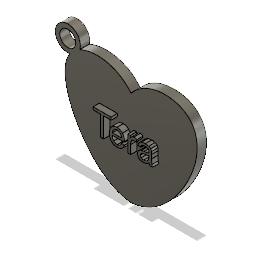
心挂件 (Autodesk Fusion 360 design; units mm, degrees)
Autodesk Fusion 360 part; units mm, degrees
sketch "草图15" plane through (0, 0, 0) normal (0, 0, 1) x (1, 0, 0)
  spline S0 degree 5 poles (0, 25) (-0.3399, 25.4215) (-1.0493, 26.2218) (-2.2021, 27.2937) (-3.9173, 28.4651) (-6.346, 29.4886) (-9.0135, 30.049) (-11.8244, 30.1104) (-14.6065, 29.6188) (-17.1328, 28.5147) (-19.1721, 26.7575) (-20.5275, 24.3447) (-21.0876, 21.3391) (-20.8505, 17.8796) (-19.8871, 14.1498) (-18.3175, 10.3575) (-16.2836, 6.7096) (-13.9259, 3.3912) (-11.3559, 0.5375) (-8.6457, -1.7723) (-5.8398, -3.4971) (-3.5364, -4.3975) (-1.7796, -4.8031) (-0.5953, -4.9543) (0, -5) knots 0 0 0 0 0 0 0.05 0.1 0.15 0.2 0.25 0.3 0.35 0.4 0.45 0.5 0.55 0.6 0.65 0.7 0.75 0.8 0.85 0.9 0.95 1 1 1 1 1 1
  spline S1 degree 5 poles (0, 25) (0.3399, 25.4215) (1.0493, 26.2218) (2.2021, 27.2937) (3.9173, 28.4651) (6.346, 29.4886) (9.0135, 30.049) (11.8244, 30.1104) (14.6065, 29.6188) (17.1328, 28.5147) (19.1721, 26.7575) (20.5275, 24.3447) (21.0876, 21.3391) (20.8505, 17.8796) (19.8871, 14.1498) (18.3175, 10.3575) (16.2836, 6.7096) (13.9259, 3.3912) (11.3559, 0.5375) (8.6457, -1.7723) (5.8398, -3.4971) (3.5364, -4.3975) (1.7796, -4.8031) (0.5953, -4.9543) (0, -5) knots 0 0 0 0 0 0 0.05 0.1 0.15 0.2 0.25 0.3 0.35 0.4 0.45 0.5 0.55 0.6 0.65 0.7 0.75 0.8 0.85 0.9 0.95 1 1 1 1 1 1
  line L0 (3.122, 21.1295) -> (-3.122, 28.8705)
  line L1 (-4.1912, -4.6775) -> (4.1912, -5.3225)
  line L2 (-3.122, 21.1295) -> (3.122, 28.8705)
  line L3 (4.1912, -4.6775) -> (-4.1912, -5.3225)
extrude "拉伸6" add sketch "草图15" along normal blind 3 makes body 1
sketch "草图16" plane through (0, 0, 3) normal (0, 0, 1) x (1, 0, 0)
  spline S0 degree 5 poles (0, 25) (-0.3399, 25.4215) (-1.0493, 26.2218) (-2.2021, 27.2937) (-3.9173, 28.4651) (-6.346, 29.4886) (-9.0135, 30.049) (-11.8244, 30.1104) (-14.6065, 29.6188) (-17.1328, 28.5147) (-19.1721, 26.7575) (-20.5275, 24.3447) (-21.0876, 21.3391) (-20.8505, 17.8796) (-19.8871, 14.1498) (-18.3175, 10.3575) (-16.2836, 6.7096) (-13.9259, 3.3912) (-11.3559, 0.5375) (-8.6457, -1.7723) (-5.8398, -3.4971) (-3.5364, -4.3975) (-1.7796, -4.8031) (-0.5953, -4.9543) (0, -5) knots 0 0 0 0 0 0 0.05 0.1 0.15 0.2 0.25 0.3 0.35 0.4 0.45 0.5 0.55 0.6 0.65 0.7 0.75 0.8 0.85 0.9 0.95 1 1 1 1 1 1
  spline S1 degree 5 poles (0, -5) (0.5953, -4.9543) (1.7796, -4.8031) (3.5364, -4.3975) (5.8398, -3.4971) (8.6457, -1.7723) (11.3559, 0.5375) (13.9259, 3.3912) (16.2836, 6.7096) (18.3175, 10.3575) (19.8871, 14.1498) (20.8505, 17.8796) (21.0876, 21.3391) (20.5275, 24.3447) (19.1721, 26.7575) (17.1328, 28.5147) (14.6065, 29.6188) (11.8244, 30.1104) (9.0135, 30.049) (6.346, 29.4886) (3.9173, 28.4651) (2.2021, 27.2937) (1.0493, 26.2218) (0.3399, 25.4215) (0, 25) knots -1 -1 -1 -1 -1 -1 -0.95 -0.9 -0.85 -0.8 -0.75 -0.7 -0.65 -0.6 -0.55 -0.5 -0.45 -0.4 -0.35 -0.3 -0.25 -0.2 -0.15 -0.1 -0.05 0 0 0 0 0 0
  line L0 (-10, 10) -> (8.7939, 10) construction
  line L1 (8.7939, 10) -> (8.7939, 20) construction
  line L2 (8.7939, 20) -> (-10, 20) construction
  line L3 (-10, 20) -> (-10, 10) construction
  text T0 "Tera" font "Arial" height 10 align ink ink in box 0 x 0 at (-10, 10) x (1, 0) y (0, 1) spacing 1 kerned height is em
extrude "拉伸7" add sketch "草图16" along normal blind 2 text T0 bodies 1
sketch "草图17" plane through (0, 0, 0) normal (0, 0, 1) x (1, 0, 0)
  circle A0 centre (-50, 20) radius 2.5
  circle A1 centre (-50, 20) radius 4
  dimension "d50" = 5
  dimension "d51" = 8
  measures "d50" diameter of A0
  measures "d51" diameter of A1
extrude "拉伸8" add sketch "草图17" along normal blind 3 separate body makes body 2
move_body "移动4" bodies 2 to x (1, 0, 0) y (0, 1, 0) z (0, 0, 1) at (30, 10, 0)
combine "合并6" operation add target body 2 tool bodies 1
sketch "草图13" plane through (0, 0, 0) normal (0, 0, 1) x (1, 0, 0)
  circle A0 centre (-24, 17) radius 40.6099
  line L0 (-26.4265, 32.3206) -> (-7.8035, 50.9437)
  line L1 (-45.8508, 38.8508) -> (-28.657, 30.0901)
  line L2 (-23.616, 30.8886) -> (-9.9709, 44.5336)
  line L3 (-49.893, 44.2774) -> (-26.4265, 32.3206)
  line L4 (-9.9709, 44.5336) -> (-12.9896, 25.4742)
  line L5 (-23.616, 30.8886) -> (-12.9896, 25.4742)
  line L6 (-10.1791, 24.0421) -> (13.2874, 12.0854)
  line L7 (-6.059, 50.0549) -> (-10.1791, 24.0421)
  line L8 (-25.8465, 28.6581) -> (-13.4831, 22.3586)
  line L9 (-10.6725, 20.9266) -> (6.5212, 12.1659)
  line L10 (-10.6725, 20.9266) -> (-12.5382, 9.1472)
  line L11 (-13.0316, 6.0316) -> (-17.1517, -19.9811)
  line L12 (-13.4831, 22.3586) -> (-15.6537, 8.6537)
  line L13 (-16.1472, 5.5382) -> (-19.1659, -13.5212)
  line L14 (6.5212, 12.1659) -> (-12.5382, 9.1472)
  line L15 (12.9811, 10.1517) -> (-13.0316, 6.0316)
  line L16 (-27.9266, 3.6725) -> (-19.1659, -13.5212)
  line L17 (-15.6537, 8.6537) -> (-29.3586, 6.4831)
  line L18 (-32.4742, 5.9896) -> (-51.5336, 2.9709)
  line L19 (-31.0421, 3.1791) -> (-19.0854, -20.2874)
  line L20 (-16.1472, 5.5382) -> (-27.9266, 3.6725)
  line L21 (-31.0421, 3.1791) -> (-57.0549, -0.941)
  line L22 (-57.9437, 0.8035) -> (-39.3206, 19.4265)
  line L23 (-37.0901, 21.657) -> (-28.657, 30.0901)
  line L24 (-51.2774, 42.893) -> (-39.3206, 19.4265)
  line L25 (-37.8886, 16.616) -> (-32.4742, 5.9896)
  line L26 (-45.8508, 38.8508) -> (-37.0901, 21.657)
  line L27 (-35.6581, 18.8465) -> (-29.3586, 6.4831)
  line L28 (-51.5336, 2.9709) -> (-37.8886, 16.616)
  line L29 (-35.6581, 18.8465) -> (-25.8465, 28.6581)
  arc A1 (-7.8035, 50.9437) -> (-49.893, 44.2774) centre (-24, 17) ccw
  arc A2 (13.2874, 12.0854) -> (-6.059, 50.0549) centre (-24, 17) ccw
  arc A3 (-17.1517, -19.9811) -> (12.9811, 10.1517) centre (-24, 17) ccw
  arc A4 (-51.2774, 42.893) -> (-57.9437, 0.8035) centre (-24, 17) ccw
  arc A5 (-57.0549, -0.941) -> (-19.0854, -20.2874) centre (-24, 17) ccw
extrude "拉伸4" [rolled back] along distance 5 taper angle 0
sketch "草图14" plane through (0, 0, 0) normal (0, 0, 1) x (1, 0, 0)
  circle A0 centre (50, 15) radius 2.5
  circle A1 centre (50, 15) radius 4
  dimension "d36" = 5
  dimension "d37" = 8
  measures "d36" diameter of A0
  measures "d37" diameter of A1
extrude "拉伸5" [rolled back] along distance 5 taper angle 0
move_body "移动2" [rolled back] translate x -75 translate y 45 translate z 0
move_body "移动3" [rolled back] translate x 21 translate y -4 translate z 0
combine "合并5" [rolled back]
sketch "草图11" plane through (0, 0, 0) normal (0, 0, 1) x (1, 0, 0)
  line L0 (-50, 25) -> (0, 25)
  line L1 (0, 25) -> (0, 5)
  line L2 (0, 5) -> (-50, 5)
  line L3 (-50, 5) -> (-50, 25)
  arc A0 (-50, 25) -> (-50, 5) centre (-51.9859, 15) ccw
  arc A1 (-50, 22.4346) -> (-50, 7.5654) centre (-51.9859, 15) ccw
extrude "拉伸2" [rolled back] along distance 3 taper angle 0
extrude "拉伸1" [rolled back] along distance 3 taper angle 0
sketch "草图12" plane through (0, 0, 3) normal (0, 0, 1) x (1, 0, 0)
  line L0 (-50, 5) -> (0, 5)
  line L1 (0, 5) -> (0, 25)
  line L2 (0, 25) -> (-50, 25)
  line L3 (-50, 25) -> (-50, 5)
  line L4 (-35, 12) -> (-16.2061, 12) construction
  line L5 (-16.2061, 12) -> (-16.2061, 22) construction
  line L6 (-16.2061, 22) -> (-35, 22) construction
  line L7 (-35, 22) -> (-35, 12) construction
extrude "拉伸3" [rolled back] along distance 2 taper angle 0
combine "合并4" [rolled back]
